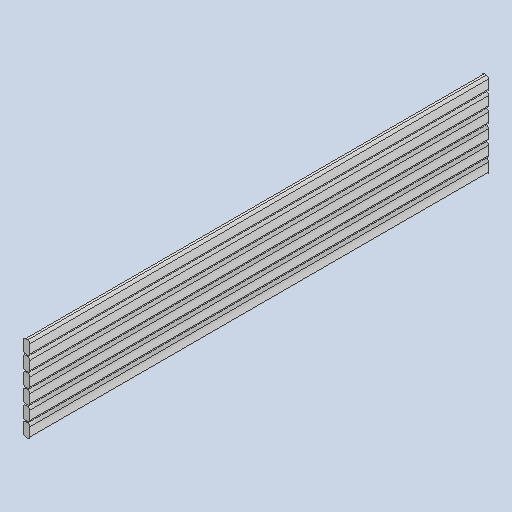
# Autodesk Inventor part: bench-slats
Saved by Autodesk Inventor 2023 (Build 270158030, 158C)
## iProperties
Created: 2024-09-09
Part Number: bench-slats
Material: Generic
Document SubType Name: Modeling
Designer: Imogen Heard
Density: 1 g/cm^3
Appearance: Default
Author: Imogen Heard
Autodesk Inventor part; units mm, degrees
ref_plane "YZ Plane" through (0, 0, 0) normal (1, 0, 0) x (0, 1, 0)
ref_plane "XZ Plane" through (0, 0, 0) normal (0, 1, 0) x (-1, 0, 0)
ref_plane "XY Plane" through (0, 0, 0) normal (0, 0, 1) x (1, 0, 0)
sketch "Sketch1" plane through (0, 0, 0) normal (0, 0, 1) x (1, 0, 0)
  arc A0 (-195, 10) -> (-205, 20) centre (-205, 10) ccw projected
  line L0 (-195, 10) -> (-195, -30) projected
  arc A1 (-205, -40) -> (-195, -30) centre (-205, -30) ccw projected
  line L1 (-205, -40) -> (-215, -40) projected
  arc A2 (-225, -30) -> (-215, -40) centre (-215, -30) ccw projected
  line L2 (-225, -30) -> (-225, 10) projected
  arc A3 (-215, 20) -> (-225, 10) centre (-215, 10) ccw projected
  line L3 (-215, 20) -> (-205, 20) projected
  arc A4 (-195, 205) -> (-205, 215) centre (-205, 205) ccw projected
  line L4 (-195, 205) -> (-195, 165) projected
  arc A5 (-205, 155) -> (-195, 165) centre (-205, 165) ccw projected
  line L5 (-205, 155) -> (-215, 155) projected
  arc A6 (-225, 165) -> (-215, 155) centre (-215, 165) ccw projected
  line L6 (-225, 165) -> (-225, 205) projected
  arc A7 (-215, 215) -> (-225, 205) centre (-215, 205) ccw projected
  line L7 (-215, 215) -> (-205, 215) projected
  arc A8 (-195, -55) -> (-205, -45) centre (-205, -55) ccw projected
  line L8 (-195, -55) -> (-195, -95) projected
  arc A9 (-205, -105) -> (-195, -95) centre (-205, -95) ccw projected
  line L9 (-205, -105) -> (-215, -105) projected
  arc A10 (-225, -95) -> (-215, -105) centre (-215, -95) ccw projected
  line L10 (-225, -95) -> (-225, -55) projected
  arc A11 (-215, -45) -> (-225, -55) centre (-215, -55) ccw projected
  line L11 (-215, -45) -> (-205, -45) projected
  arc A12 (-195, 75) -> (-205, 85) centre (-205, 75) ccw projected
  line L12 (-195, 75) -> (-195, 35) projected
  arc A13 (-205, 25) -> (-195, 35) centre (-205, 35) ccw projected
  line L13 (-205, 25) -> (-215, 25) projected
  arc A14 (-225, 35) -> (-215, 25) centre (-215, 35) ccw projected
  line L14 (-225, 35) -> (-225, 75) projected
  arc A15 (-215, 85) -> (-225, 75) centre (-215, 75) ccw projected
  line L15 (-215, 85) -> (-205, 85) projected
  arc A16 (-195, 140) -> (-205, 150) centre (-205, 140) ccw projected
  line L16 (-195, 140) -> (-195, 100) projected
  arc A17 (-205, 90) -> (-195, 100) centre (-205, 100) ccw projected
  line L17 (-205, 90) -> (-215, 90) projected
  arc A18 (-225, 100) -> (-215, 90) centre (-215, 100) ccw projected
  line L18 (-225, 100) -> (-225, 140) projected
  arc A19 (-215, 150) -> (-225, 140) centre (-215, 140) ccw projected
  line L19 (-215, 150) -> (-205, 150) projected
  arc A20 (-195, -120) -> (-205, -110) centre (-205, -120) ccw projected
  line L20 (-195, -120) -> (-195, -160) projected
  arc A21 (-205, -170) -> (-195, -160) centre (-205, -160) ccw projected
  line L21 (-205, -170) -> (-215, -170) projected
  arc A22 (-225, -160) -> (-215, -170) centre (-215, -160) ccw projected
  line L22 (-225, -160) -> (-225, -120) projected
  arc A23 (-215, -110) -> (-225, -120) centre (-215, -120) ccw projected
  line L23 (-215, -110) -> (-205, -110) projected
  line L24 (-165, 225) -> (-165, -91.0685) projected
  line L25 (-235, 225) -> (-165, 225) projected
  line L26 (-235, -175) -> (-235, 225) projected
  line L27 (-165, -225) -> (-229.3032, -225) projected
  line L28 (-165, -176.5227) -> (-165, -225) projected
  line L29 (165, 54.5458) -> (-165, -176.5227) projected
  line L30 (165, -190) -> (165, 54.5458) projected
  line L31 (235, -190) -> (165, -190) projected
  line L32 (235, 190) -> (235, -190) projected
  line L33 (165, 190) -> (235, 190) projected
  line L34 (165, 140) -> (165, 190) projected
  line L35 (-165, -91.0685) -> (165, 140) projected
  line L36 (-235, -175) -> (-685, -278.8907) projected
  line L37 (-685, -278.8907) -> (-673.7524, -327.6092) projected
  line L38 (-673.7524, -327.6092) -> (-229.3032, -225) projected
  point P0 (0, 0)
extrude "Extrusion1" add sketch "Sketch1" along normal blind 2000 and the other way blind 75 contours L0 A1 L1 A2 L2 A3 L3 A0 | L4 A5 L5 A6 L6 A7 L7 A4 | L8 A9 L9 A10 L10 A11 L11 A8 | L12 A13 L13 A14 L14 A15 L15 A12 | L16 A17 L17 A18 L18 A19 L19 A16 | L20 A21 L21 A22 L22 A23 L23 A20
